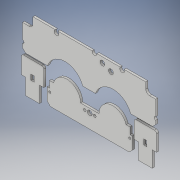
# Autodesk Inventor part: Controller_PCB_shape
Saved by Autodesk Inventor 2019 (Build 230136000, 136)
## iProperties
Created: 2019-05-10
Part Number: Controller_PCB_shape
Material: Generic
Document SubType Name: Modeling
Designer: cutla
Density: 1 g/cm^3
Appearance: Default
Author: cutla
Autodesk Inventor part; units mm, degrees
ref_plane "YZ Plane" through (0, 0, 0) normal (1, 0, 0) x (0, 1, 0)
ref_plane "XZ Plane" through (0, 0, 0) normal (0, 1, 0) x (-1, 0, 0)
ref_plane "XY Plane" through (0, 0, 0) normal (0, 0, 1) x (1, 0, 0)
sketch "Sketch1" plane through (0, 0, 0) normal (0, 0, 1) x (1, 0, 0)
  line L0 (37.6359, -48.2495) -> (-36.3641, -48.2495)
  line L1 (-39.3641, -45.2495) -> (-39.3641, -33.7495)
  line L2 (-39.3641, -33.7495) -> (-37.1141, -33.7495)
  line L3 (-37.1141, -33.7495) -> (-37.1141, -27.4995)
  line L4 (9.2609, -31.2495) -> (-7.9891, -31.2495)
  arc A0 (-7.9891, -31.2495) -> (-33.4365, -27.4995) centre (-20.9891, -31.2495) ccw
  line L5 (-37.1141, -27.4995) -> (-33.4365, -27.4995)
  circle A1 centre (-36.8641, -36.7495) radius 1
  circle A2 centre (0.6359, -34.9995) radius 2.25
  circle A3 centre (-4.0641, -34.9995) radius 1.25
  line L6 (0, 13.6122) -> (0, -36.0241) construction
  line L7 (40.6359, -45.2495) -> (40.6359, -33.7495)
  line L8 (40.6359, -33.7495) -> (38.3859, -33.7495)
  line L9 (38.3859, -33.7495) -> (38.3859, -27.4995)
  arc A4 (34.7083, -27.4995) -> (9.2609, -31.2495) centre (22.2609, -31.2495) ccw
  line L10 (38.3859, -27.4995) -> (34.7083, -27.4995)
  circle A5 centre (38.1359, -36.7495) radius 1
  circle A6 centre (5.3359, -34.9995) radius 1.25
  line L11 (44.2622, -18.6747) -> (61.2622, -18.6747)
  line L12 (63.2622, -20.6747) -> (63.2622, -35.6747)
  line L13 (42.2622, -35.6747) -> (42.2622, -20.6747)
  line L14 (59.2622, -35.6747) -> (59.2622, -50.6747)
  line L15 (59.2622, -50.6747) -> (46.2622, -50.6747)
  line L16 (46.2622, -50.6747) -> (46.2622, -35.6747)
  arc A7 (44.2622, -18.6747) -> (42.2622, -20.6747) centre (44.2622, -20.6747) ccw
  arc A8 (63.2622, -20.6747) -> (61.2622, -18.6747) centre (61.2622, -20.6747) ccw
  line L17 (42.2622, -35.6747) -> (46.2622, -35.6747)
  line L18 (59.2622, -35.6747) -> (63.2622, -35.6747)
  line L19 (51.2622, -30.6747) -> (54.2622, -30.6747)
  line L20 (54.2622, -30.6747) -> (54.2622, -35.6747)
  line L21 (54.2622, -35.6747) -> (51.2622, -35.6747)
  line L22 (51.2622, -35.6747) -> (51.2622, -30.6747)
  line L23 (-61.5722, -19.0079) -> (-44.5722, -19.0079)
  line L24 (-42.5722, -21.0079) -> (-42.5722, -36.0079)
  line L25 (-63.5722, -36.0079) -> (-63.5722, -21.0079)
  line L26 (-46.5722, -36.0079) -> (-46.5722, -51.0079)
  line L27 (-46.5722, -51.0079) -> (-59.5722, -51.0079)
  line L28 (-59.5722, -51.0079) -> (-59.5722, -36.0079)
  arc A9 (-61.5722, -19.0079) -> (-63.5722, -21.0079) centre (-61.5722, -21.0079) ccw
  arc A10 (-42.5722, -21.0079) -> (-44.5722, -19.0079) centre (-44.5722, -21.0079) ccw
  line L29 (-63.5722, -36.0079) -> (-59.5722, -36.0079)
  line L30 (-46.5722, -36.0079) -> (-42.5722, -36.0079)
  line L31 (-54.5722, -31.0079) -> (-51.5722, -31.0079)
  line L32 (-51.5722, -31.0079) -> (-51.5722, -36.0079)
  line L33 (-51.5722, -36.0079) -> (-54.5722, -36.0079)
  line L34 (-54.5722, -36.0079) -> (-54.5722, -31.0079)
  arc A11 (39.0284, -16.5) -> (5.9716, -16.5) centre (22.5, -22.25) ccw
  arc A12 (-5.9716, -16.5) -> (-39.0284, -16.5) centre (-22.5, -22.25) ccw
  arc A13 (-31.6589, 16.5) -> (-29.3411, 16.5) centre (-30.5, 14.5714) ccw
  circle A14 centre (12.5, 11.5) radius 2.25
  circle A15 centre (20.5, 8.5) radius 2.25
  arc A16 (29.1535, 16.5) -> (32.8465, 16.5) centre (31, 15.2143) ccw
  arc A17 (2.766, 16.5) -> (7.234, 16.5) centre (5, 16.2321) ccw
  line L35 (-39.0284, -16.5) -> (-59.5, -16.5)
  line L36 (59.5, -16.5) -> (39.0284, -16.5)
  line L37 (5.9716, -16.5) -> (-5.9716, -16.5)
  line L38 (-52.6712, 16.5) -> (-31.6589, 16.5)
  line L39 (-29.3411, 16.5) -> (2.766, 16.5)
  line L40 (7.234, 16.5) -> (29.1535, 16.5)
  line L41 (32.8465, 16.5) -> (53.1712, 16.5)
  line L42 (-62.5, 7.0455) -> (-56.1712, 7.0455)
  line L43 (-52.6712, 10.5455) -> (-52.6712, 16.5)
  arc A18 (-56.1712, 7.0455) -> (-52.6712, 10.5455) centre (-56.1712, 10.5455) ccw
  line L44 (62.5, 7.0455) -> (56.6712, 7.0455)
  line L45 (53.1712, 10.5455) -> (53.1712, 16.5)
  arc A19 (53.1712, 10.5455) -> (56.6712, 7.0455) centre (56.6712, 10.5455) ccw
  line L46 (-39.3641, -45.2495) -> (-36.3641, -48.2495)
  line L47 (37.6359, -48.2495) -> (40.6359, -45.2495)
  arc A20 (62.5, -7) -> (62.5, -10) centre (62.5, -8.5) ccw
  line L48 (62.5, -13.5) -> (59.5, -16.5)
  line L49 (-59.5, -16.5) -> (-62.5, -13.5)
  line L50 (62.5, -13.5) -> (62.5, -10)
  line L51 (62.5, -7) -> (62.5, 7.0455)
  arc A21 (-62.5, -10) -> (-62.5, -7) centre (-62.5, -8.5) ccw
  line L52 (-62.5, 7.0455) -> (-62.5, -7)
  line L53 (-62.5, -10) -> (-62.5, -13.5)
  point P0 (0, 0)
  point P1 (40.6359, -48.2495)
  point P2 (-39.3641, -48.2495)
  point P3 (0.6359, -48.2495)
  point P4 (0.6359, -31.2495)
  point P5 (63.2622, -18.6747)
  point P6 (52.7622, -18.6747)
  point P7 (52.7622, -35.6747)
  point P8 (52.7622, -35.6747)
  point P9 (52.7622, -30.6747)
  point P10 (-42.5722, -19.0079)
  point P11 (-53.0722, -19.0079)
  point P12 (-53.0722, -36.0079)
  point P13 (-53.0722, -36.0079)
  point P14 (-53.0722, -31.0079)
  point P15 (62.5, -16.5)
  point P16 (-62.5, -16.5)
  point P17 (-62.5, 0)
  point P18 (0, -16.5)
  point P19 (-62.5, -12.5)
  point P20 (-58.5, -16.5)
  point P21 (-62.5, -16.5)
  point P22 (58.5, -16.5)
  point P23 (62.5, -16.5)
  point P24 (-62.5, -16.5)
  dimension "d0" = 80
  dimension "d1" = 14.5
  dimension "d3" = 2.25
  dimension "d4" = 6.25
  dimension "d5" = 17.25
  dimension "d6" = 17
  dimension "d7" = 26
  dimension "d8" = 2
  dimension "d9" = 2.5
  dimension "d11" = 2.5
  dimension "d12" = 1.5
  dimension "d13" = 1.2
  dimension "d14" = 3
  dimension "d16" = 17
  dimension "d17" = 13
  dimension "d18" = 15
  dimension "d19" = 2
  dimension "d20" = 3
  dimension "d21" = 5
  dimension "d22" = 17
  dimension "d23" = 13
  dimension "d24" = 15
  dimension "d25" = 2
  dimension "d26" = 3
  dimension "d27" = 5
  dimension "d30" = 35
  dimension "d31" = 35
  dimension "d32" = 45
  dimension "d33" = 22.5
  dimension "d35" = 4.5
  dimension "d36" = 4.5
  dimension "d37" = 4.5
  dimension "d38" = 4.5
  dimension "d39" = 4.5
  dimension "d64" = 1.2
  dimension "d65" = 3.75
  dimension "d66" = 2.5
  dimension "d67" = 4.5
  dimension "d74" = 3
  dimension "d75" = 3
  dimension "d76" = 3
  dimension "d77" = 3
  dimension "d78" = 8
  dimension "d95" = 3
  dimension "d96" = 8
  dimension "d97" = 3
  dimension "d98" = 3
  dimension "d99" = 3
  dimension "d100" = 3
  dimension "d102" = 2.5
  constraints: 108 end point, 30 point on circle, 22 centre point, 16 point on line, 7 midpoint, 3 symmetric about line, 2 horizontal, 2 vertical, 1 other
  measures "d0" distance of point (40.636, -48.249) point (-39.364, -48.249)
  measures "d1" distance of point (-39.364, -48.249) L1.end
  measures "d3" distance of L1.end L2.end
  measures "d4" distance of L2.end L3.end
  measures "d5" distance of L4.start L4.end
  measures "d6" distance between parallel lines of L0 L4
  measures "d7" diameter of A0
  measures "d8" diameter of A1
  measures "d9" distance from line of L1 A1.centre
  measures "d11" diameter of A3
  measures "d12" distance edge to line of A2 L4
  measures "d14" distance from line of L2 A1.centre
  measures "d16" distance of point (63.262, -18.675) L12.end
  measures "d17" distance of L14.end L15.end
  measures "d18" distance of L14.start L14.end
  measures "d19" radius of A7
  measures "d20" distance of L20.end L21.end
  measures "d21" distance of L19.end L20.end
  measures "d22" distance of point (-42.572, -19.008) L30.end
  measures "d23" distance of L27.start L27.end
  measures "d24" distance of L30.start L27.start
  measures "d25" radius of A9
  measures "d26" distance of L32.end L34.start
  measures "d27" distance of L31.end L32.end
  measures "d30" diameter of A11
  measures "d31" diameter of A12
  measures "d32" distance of A11.centre A12.centre
  measures "d33" distance from line of L6 A11.centre
  measures "d35" diameter of A13
  measures "d36" diameter of A14
  measures "d37" diameter of A15
  measures "d38" diameter of A16
  measures "d39" diameter of A17
  measures "d65" distance of point (0.636, -31.249) A2.centre
  measures "d66" diameter of A6
  measures "d67" diameter of A2
  measures "d74" distance of L1.start point (-39.364, -48.249)
  measures "d75" distance of L0.end point (-39.364, -48.249)
  measures "d76" distance of L0.start point (40.636, -48.249)
  measures "d77" distance of L7.start point (40.636, -48.249)
  measures "d78" distance from line of L40 A15.centre
  measures "d95" diameter of A20
  measures "d96" distance from line of A20.centre L36
  measures "d97" distance of L48.start point (62.5, -16.5)
  measures "d98" distance of L36.start point (62.5, -16.5)
  measures "d99" distance of L35.end point (-62.5, -16.5)
  measures "d100" distance of L49.end point (-62.5, -16.5)
  measures "d102" distance from line of L7 A5.centre
extrude "Extrusion1" add sketch "Sketch1" along normal blind 2
body "Solid1"
